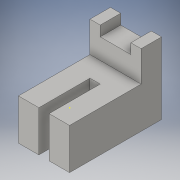
# Autodesk Inventor part: Unit 7.1
Saved by Autodesk Inventor 2016 (Build 200138000, 138)
## iProperties
Created: 2017-03-02
Part Number: Unit 7.1
Material: Generic
Document SubType Name: Modeling
Designer: 196918
Mass: 56.3305 g
Surface Area: 95.9676 cm^2
Volume: 56.3305 cm^3
Density: 1 g/cm^3
Appearance: Default
Author: 196918
Autodesk Inventor part; units mm, degrees
ref_plane "YZ Plane" through (0, 0, 0) normal (1, 0, 0) x (0, 1, 0)
ref_plane "XZ Plane" through (0, 0, 0) normal (0, 1, 0) x (-1, 0, 0)
ref_plane "XY Plane" through (0, 0, 0) normal (0, 0, 1) x (1, 0, 0)
sketch "Sketch1" plane through (0, 0, 0) normal (0, 1, 0) x (-1, 0, 0)
  line L0 (-9.3834, 9.4925) -> (22.3666, 9.4925)
  line L1 (22.3666, 9.4925) -> (22.3666, -47.6575)
  line L2 (22.3666, -47.6575) -> (-9.3834, -47.6575)
  line L3 (-9.3834, -47.6575) -> (-9.3834, 9.4925)
  point P0 (0, 0)
  dimension "d0" = 31.75
  dimension "d1" = 57.15
  constraints: 8 end point, 2 parallel, 1 horizontal, 1 perpendicular
  measures "d0" distance of L1.end L2.end
  measures "d1" distance of L0.end L1.end
extrude "Extrusion1" add sketch "Sketch1" along normal blind 25.4
sketch "Sketch2" plane through (0, 25.4, 0) normal (0, 1, 0) x (1, 0, 0)
  point P0 (0, 0)
sketch "Sketch3" plane through (0, 25.4, 0) normal (0, 1, 0) x (1, 0, 0)
  line L0 (-22.3666, -9.4925) -> (9.3834, -9.4925) construction
  line L1 (-22.3666, -9.4925) -> (-9.6666, -9.4925) construction
  line L2 (9.3834, -9.4925) -> (-3.3166, -9.4925) construction
  line L3 (-9.6666, -9.4925) -> (-3.3166, -9.4925) construction
  line L4 (-3.3166, -9.4925) -> (-3.3166, 22.2575)
  line L5 (-3.3166, 22.2575) -> (-9.6666, 22.2575)
  line L6 (-9.6666, 22.2575) -> (-9.6666, -9.4925)
  line L7 (-9.6666, -9.4925) -> (-3.3166, -9.4925)
  point P0 (0, 0)
  dimension "d4" = 12.7
  dimension "d5" = 12.7
  dimension "d6" = 31.75
  constraints: 14 end point, 2 parallel, 2 point on line, 1 collinear, 1 horizontal, 1 perpendicular
  measures "d4" distance of L0.start L1.end
  measures "d5" distance of L0.end L2.end
  measures "d6" distance of L4.end L3.end
extrude "Extrusion2" cut sketch "Sketch3" against normal blind 25.4
sketch "Sketch4" plane through (0, 25.4, 0) normal (0, 1, 0) x (1, 0, 0)
  line L0 (9.3834, 47.6575) -> (9.3834, -9.4925) projected
  line L1 (-22.3666, 47.6575) -> (9.3834, 47.6575)
  line L2 (9.3834, 47.6575) -> (9.3834, 34.9575)
  line L3 (9.3834, 34.9575) -> (-22.3666, 34.9575)
  line L4 (-22.3666, 34.9575) -> (-22.3666, 47.6575)
  point P0 (0, 0)
  dimension "d9" = 12.7
  constraints: 8 end point, 2 parallel, 1 horizontal, 1 perpendicular, 1 point on line
  measures "d9" distance of L1.end L2.end
extrude "Extrusion3" add sketch "Sketch4" along normal blind 12.7
sketch "Sketch5" plane through (0, 38.1, 0) normal (0, 1, 0) x (1, 0, 0)
  line L0 (9.3834, 34.9575) -> (-22.3666, 34.9575) projected
  line L1 (-22.3666, 47.6575) -> (9.3834, 47.6575) projected
  line L2 (9.3834, 34.9575) -> (3.0334, 34.9575)
  line L3 (3.0334, 34.9575) -> (3.0334, 47.6575)
  line L4 (3.0334, 47.6575) -> (9.3834, 47.6575)
  line L5 (9.3834, 47.6575) -> (9.3834, 34.9575)
  line L6 (-22.3666, 47.6575) -> (-16.0166, 47.6575)
  line L7 (-16.0166, 47.6575) -> (-16.0166, 34.9575)
  line L8 (-16.0166, 34.9575) -> (-22.3666, 34.9575)
  line L9 (-22.3666, 34.9575) -> (-22.3666, 47.6575)
  point P0 (0, 0)
  dimension "d12" = 6.35
  dimension "d13" = 6.35
  constraints: 16 end point, 4 parallel, 2 horizontal, 2 perpendicular, 2 point on line
  measures "d12" distance of L3.end L4.end
  measures "d13" distance of L7.end L8.end
extrude "Extrusion4" add sketch "Sketch5" along normal blind 6.35 contours L0 L3 L1 L5 | L0 L9 L1 L7
body "Solid1"
